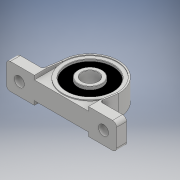
# Autodesk Inventor part: kp08
Saved by Autodesk Inventor 2018 (Build 220112000, 112)
## iProperties
Created: 2018-09-20
Part Number: kp08
Material: Genérico
Document SubType Name: Modeling
Designer: Georgines
Density: 1 g/cm^3
Appearance: Padrão
Author: Georgines
Autodesk Inventor part; units mm, degrees
ref_plane "YZ Plane" through (0, 0, 0) normal (1, 0, 0) x (0, 1, 0)
ref_plane "XZ Plane" through (0, 0, 0) normal (0, 1, 0) x (-1, 0, 0)
sketch "Esboço1" plane through (0, 0, 0) normal (0, 0, 1) x (1, 0, 0)
  circle A0 centre (0, 0) radius 13.5
  line L0 (-27.5, -14.25) -> (27.5, -14.25)
  line L1 (0, 25.3783) -> (0, -25.3783) construction
  line L2 (-27.5, -9.25) -> (-27.5, -14.25)
  line L3 (27.5, -9.25) -> (27.5, -14.25)
  line L4 (-27.5, -9.25) -> (-15.25, -9.25)
  line L5 (15.25, -9.25) -> (27.5, -9.25)
  line L6 (-14.25, 0) -> (-14.25, -8.25)
  line L7 (14.25, 0) -> (14.25, -8.25)
  arc A1 (14.25, -8.25) -> (15.25, -9.25) centre (15.25, -8.25) ccw
  arc A2 (-15.25, -9.25) -> (-14.25, -8.25) centre (-15.25, -8.25) ccw
  arc A3 (14.25, 0) -> (-14.25, 0) centre (0, 0) ccw
  point P0 (0, -14.25)
  point P1 (-10.8397, -9.25)
  point P2 (10.8397, -9.25)
  dimension "d1" = 27
  dimension "d5" = 55
  dimension "d6" = 5
  dimension "d7" = 1
  dimension "d8" = 1
  constraints: 16 end point, 6 point on circle, 6 tangent, 4 centre point, 4 perpendicular, 3 coincident, 3 point on line, 3 vertical, 2 midpoint, 1 horizontal
  measures "d1" diameter of A0
  measures "d5" distance of L0.start L0.end
  measures "d6" distance of L2.start L0.start
  measures "d7" radius of A1
  measures "d8" radius of A2
extrude "Extrusão1" add sketch "Esboço1" along normal blind 13
sketch "Esboço2" plane through (27.5, -14.25, 0) normal (1, 0, 0) x (0, 0, -1)
  line L0 (-13.0565, 6) -> (-11.897, 14.25)
  line L1 (0, 14.25) -> (-13, 14.25) projected
  line L2 (0, 6) -> (-13, 6) projected
  line L3 (0, 6) -> (-1.1683, 14.3128)
  line L4 (-1.1683, 14.3128) -> (-1.1683, 28.5)
  line L5 (0, 28.5) -> (-13, 28.5) projected
  line L6 (-11.897, 14.25) -> (-11.897, 28.5)
  line L7 (0, 27.75) -> (-13, 27.75) projected
  line L8 (-11.897, 28.5) -> (-16.0762, 28.5)
  line L9 (-16.0762, 28.5) -> (-16.0762, 6)
  line L10 (-16.0762, 6) -> (-13.0565, 6)
  line L11 (-1.1683, 28.5) -> (3.8166, 28.5)
  line L12 (3.8166, 28.5) -> (3.8166, 6)
  line L13 (3.8166, 6) -> (0, 6)
  dimension "d11" = 98
  dimension "d12" = 98
  constraints: 20 end point, 5 perpendicular, 4 point on line, 2 vertical, 1 parallel
  measures "d11" angle of L3 L1
  measures "d12" angle of L1 L0
extrude "Extrusão2" cut sketch "Esboço2" against normal through all contours L10 L9 L8 L5 L6 L0 | L3 L4 L5 L11 L12 L13
ref_plane "Plano de trabalho1" through (0, 0, 11.5) normal (0, 0, 1) x (1, 0, 0)
sketch "Esboço3" plane through (0, 0, 11.5) normal (0, 0, 1) x (1, 0, 0)
  circle A0 centre (0, 0) radius 13.5
  constraints: 1 centre point, 1 coincident
extrude "Extrusão3" add sketch "Esboço3" against normal blind 10
sketch "Esboço4" plane through (0, 0, 1.5) normal (0, 0, -1) x (-1, 0, 0)
  circle A0 centre (0, 0) radius 11.5
  dimension "d19" = 23
  constraints: 1 centre point, 1 coincident
  measures "d19" diameter of A0
extrude "Extrusão4" cut sketch "Esboço4" against normal blind 1
sketch "Esboço5" plane through (0, 0, 11.5) normal (0, 0, 1) x (1, 0, 0)
  circle A0 centre (0, 0) radius 11.5
  dimension "d22" = 23
  constraints: 1 centre point, 1 coincident
  measures "d22" diameter of A0
extrude "Extrusão5" cut sketch "Esboço5" against normal blind 1
sketch "Esboço6" plane through (0, 0, 2.5) normal (0, 0, -1) x (-1, 0, 0)
  circle A0 centre (0, 0) radius 6
  dimension "d25" = 12
  constraints: 1 centre point, 1 coincident
  measures "d25" diameter of A0
extrude "Extrusão6" add sketch "Esboço6" along normal blind 3
sketch "Esboço7" plane through (0, 0, 10.5) normal (0, 0, 1) x (1, 0, 0)
  circle A0 centre (0, 0) radius 6
  dimension "d28" = 12
  constraints: 1 centre point, 1 coincident
  measures "d28" diameter of A0
extrude "Extrusão7" add sketch "Esboço7" along normal blind 1.5
sketch "Esboço8" plane through (0, 0, -0.5) normal (0, 0, -1) x (-1, 0, 0)
  circle A0 centre (0, 0) radius 4
  dimension "d31" = 8
  constraints: 1 centre point, 1 coincident
  measures "d31" diameter of A0
hole "Furo1" at (0, 0, -0.5) direction (0, 0, 1) diameter 8 end through all
fillet "Arredondamento1" radius 2 4 edges at (-27.5, -11.75, 13) (-27.5, -11.75, 0) (27.5, -11.75, 0) (27.5, -11.75, 13)
sketch "Esboço9" plane through (0, 0, 13) normal (0, 0, 1) x (1, 0, 0)
  arc A0 (-13.4999, -0.0397) -> (13.5, 0) centre (0, 0) ccw
  line L0 (-13.4999, -0.0397) -> (-13.4999, -14.25)
  line L1 (14.25, -8.25) -> (14.25, 0) projected
  line L2 (-13.4999, -14.25) -> (13.5, -14.25)
  line L3 (-25.5, -14.25) -> (25.5, -14.25) projected
  arc A1 (10.6859, -8.25) -> (13.4999, 0.0628) centre (0, 0) ccw projected
  line L4 (13.5, 0) -> (13.5, -14.25)
  circle A2 centre (0, 0) radius 13.5
  dimension "d40" = 27
  constraints: 6 end point, 3 point on circle, 2 centre point, 2 tangent, 1 coincident, 1 perpendicular, 1 point on line, 1 vertical
  measures "d40" diameter of A2
extrude "Extrusão8" cut sketch "Esboço9" against normal blind 2 contours A0 L4 L2 L0
sketch "Esboço10" plane through (0, 0, 0) normal (0, 0, -1) x (-1, 0, 0)
  arc A0 (13.4999, -0.0397) -> (13.4999, 0.0397) centre (0, 0) ccw
  line L0 (-13.5, -14.25) -> (13.4999, -14.25) projected
  line L1 (-13.5, 0) -> (-13.5, -14.25)
  line L2 (-13.5, -14.25) -> (13.4999, -14.25)
  arc A1 (-13.5, 0) -> (13.4999, -0.0397) centre (0, 0) ccw projected
  line L3 (13.4999, -14.25) -> (13.4999, -0.0397)
  circle A2 centre (0, 0) radius 13.5
  dimension "d43" = 27
  constraints: 6 end point, 2 centre point, 2 perpendicular, 2 point on circle, 1 coincident, 1 collinear, 1 point on line
  measures "d43" diameter of A2
extrude "Extrusão9" cut sketch "Esboço10" against normal blind 2 contours L3 L0 L1 A1
fillet "Arredondamento2" radius 0.2 6 edges at (-11.5, 0, 11.5) (-6, 0, 12) (0, -4, 12) (11.5, 0, 1.5) (6, 0, -0.5) (0, -4, -0.5)
sketch "Esboço11" plane through (27.5, -14.25, 2) normal (0, -1, 0) x (1, 0, 0)
  line L0 (0, 0) -> (0, 9) construction
  line L1 (0, 4.5) -> (-55, 4.5) construction
  line L2 (-55, 0) -> (-55, 9) construction
  line L3 (-40.9999, 0) -> (-14, 0) construction
  line L4 (-27.5, 0) -> (-27.5, 9.0849) construction
  circle A0 centre (-6.5, 4.5) radius 2.5 construction
  circle A1 centre (-48.5, 4.5) radius 2.5 construction
  point P0 (-27.5, -2)
  dimension "d48" = 5
  dimension "d49" = 5
  dimension "d50" = 21
  dimension "d51" = 21
  constraints: 4 end point, 3 midpoint, 2 centre point, 2 point on line, 1 vertical
  measures "d48" diameter of A0
  measures "d49" diameter of A1
  measures "d50" distance from line of L4 A0.centre
  measures "d51" distance from line of L4 A1.centre
hole "Furo2" at (21, -14.25, 6.5) at (-21, -14.25, 6.5) direction (0, 1, 0) diameter 5 end through all
equation "\"d51\" = d50"
